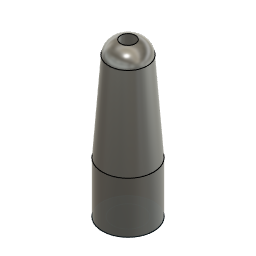
Nozzle_for_flux_dispencer (Autodesk Fusion 360 design; units mm, degrees)
Autodesk Fusion 360 part; units mm, degrees
sketch "Sketch1" plane through (0, 0, 0) normal (0, 1, 0) x (1, 0, 0)
  circle A0 centre (0, 0) radius 2
  circle A1 centre (0, 0) radius 3.5
  dimension "d1" = 4
  dimension "d2" = 7
  constraint coincident A0.centre A1.centre
  constraint concentric A0 A1
  measures "d1" diameter of A0
  measures "d2" diameter of A1
ref_plane "WorkPlane1" through (0, 14, 0) normal (0, 1, 0) x (0, 0, 1)
sketch "Sketch2" plane through (0, 14, 0) normal (0, 1, 0) x (1, 0, 0)
  circle A0 centre (0, 0) radius 0.9
  circle A1 centre (0, 0) radius 2
  dimension "d4" = 1.8
  dimension "d5" = 4
  constraint coincident A0.centre A1.centre
  measures "d4" diameter of A0
  measures "d5" diameter of A1
loft "Loft1" add profiles "Sketch1", "Sketch2" section 1 section 2 makes body 1
loft "Loft2" cut profiles "Sketch1", "Sketch2" section 1 contours A0 section 2 contours A0 bodies 1
extrude "Extrude1" add sketch "Sketch1" against normal blind 6 bodies 1
fillet "Fillet1" radius 374.5 1 edges at (-3.2631, 0, 1.2657) on bodies 1
sketch "Sketch3" plane through (0, 0, 0) normal (0, 1, 0) x (1, 0, 0)
  circle A0 centre (0, 0) radius 2.125
  circle A1 centre (0, 0) radius 3.5
  dimension "d10" = 4.25
  dimension "d11" = 7
  constraint coincident A0.centre A1.centre
  constraint concentric A0 A1
  measures "d10" diameter of A0
  measures "d11" diameter of A1
ref_plane "WorkPlane2" through (0, 14, 0) normal (0, 1, 0) x (0, 0, 1)
sketch "Sketch4" plane through (0, 14, 0) normal (0, 1, 0) x (1, 0, 0)
  circle A0 centre (0, 0) radius 1
  circle A1 centre (0, 0) radius 2.5
  dimension "d13" = 2
  dimension "d14" = 5
  constraint coincident A0.centre A1.centre
  measures "d13" diameter of A0
  measures "d14" diameter of A1
loft "Loft3" add profiles "Sketch3", "Sketch4" section 1 section 2 separate body makes body 2
loft "Loft4" cut profiles "Sketch3", "Sketch4" section 1 contours A0 section 2 contours A0 bodies 2
extrude "Extrude2" add 1 faces at (3.0207, 0, 0.2795) along direction (0, -1, 0) blind 7 on bodies 2 bodies 2
fillet "Fillet2" radius 2 1 edges at (-2.3308, 14, -0.904) on bodies 2
move_body "Move1" bodies 2 to x (1, 0, 0) y (0, 1, 0) z (0, 0, 1) at (0, 0, 12)
fillet "Fillet3" radius 1.5 1 edges at (-1.8647, 14, -0.7232) on bodies 1
scale "Scale1" factor 1.2 about (-2.6303, 12.176, 12) bodies 2
sketch "Sketch5" plane through (0, -10.8352, 0) normal (0, -1, 0) x (1, 0, 0)
  circle A0 centre (0.5261, 12) radius 2.55
  circle A1 centre (0.5261, 12) radius 4.2
hidden bodies 1
named bodies: "dsunykNozzle", "rmaNozzle"
